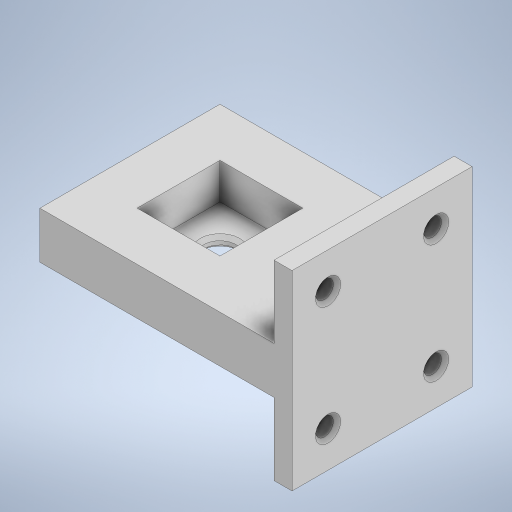
# Autodesk Inventor part: Стенка энкодер
Saved by Autodesk Inventor 2023 (Build 270158000, 158)
## iProperties
Created: 2022-05-02
Part Number: Стенка энкодер
Material: Типовые
Document SubType Name: Modeling
Designer: User
Density: 1 g/cm^3
Appearance: По умолчанию
Author: User
Autodesk Inventor part; units mm, degrees
ref_plane "YZ Plane" through (0, 0, 0) normal (1, 0, 0) x (0, 1, 0)
ref_plane "XZ Plane" through (0, 0, 0) normal (0, 1, 0) x (-1, 0, 0)
ref_plane "XY Plane" through (0, 0, 0) normal (0, 0, 1) x (1, 0, 0)
sketch "Эскиз1" plane through (0, 0, 0) normal (0, 1, 0) x (-1, 0, 0)
  line L0 (0, 0) -> (-70, 0)
  line L1 (-70, 0) -> (-70, -50)
  line L2 (-70, -50) -> (0, -50)
  line L3 (0, -50) -> (0, 0)
  line L4 (-70, 0) -> (-25, 0)
  line L5 (-25, 0) -> (-25, -25)
  line L6 (-25, -25) -> (-70, -25)
  line L7 (-70, -25) -> (-70, 0)
  circle A0 centre (-25, -25) radius 4.5
  dimension "d0" = 70
  dimension "d1" = 50
  dimension "d2" = 45
  dimension "d3" = 25
  dimension "d4" = 9
  constraints: 16 end point, 4 parallel, 2 horizontal, 2 perpendicular, 1 centre point, 1 coincident
  measures "d0" distance of L2.end L1.end
  measures "d1" distance of L1.end L0.end
  measures "d2" distance of L5.end L6.end
  measures "d3" distance of L4.end L5.end
  measures "d4" diameter of A0
extrude "Выдавливание1" add sketch "Эскиз1" along normal blind 3 contours L3 L2 L1 L6 A0 L5 L0 | L5 A0 L6 L1 L0
sketch "Эскиз2" plane through (0, 3, 0) normal (0, 1, 0) x (1, 0, 0)
  circle A0 centre (25, 25) radius 4.5 projected
  line L0 (25, 25) -> (25, 13.5)
  line L1 (25, 13.5) -> (13.5, 13.5)
  line L2 (13.5, 13.5) -> (36.5, 13.5)
  line L3 (36.5, 13.5) -> (36.5, 36.5)
  line L4 (36.5, 36.5) -> (13.5, 36.5)
  line L5 (13.5, 36.5) -> (13.5, 13.5)
  line L6 (70, 50) -> (0, 50) projected
  line L7 (0, 0) -> (70, 0)
  line L8 (70, 0) -> (70, 50)
  line L9 (70, 50) -> (0, 50)
  line L10 (0, 50) -> (0, 0)
  dimension "d7" = 11.5
  dimension "d8" = 11.5
  dimension "d9" = 23
  dimension "d10" = 23
  constraints: 20 end point, 4 parallel, 3 perpendicular, 2 horizontal, 1 vertical
  measures "d7" distance of L0.start L0.end
  measures "d8" distance of L0.end L1.end
  measures "d9" distance of L4.end L3.end
  measures "d10" distance of L3.end L2.end
extrude "Выдавливание2" add sketch "Эскиз2" along normal blind 10 contours L8 L7 L10 L6
sketch "Эскиз3" plane through (70, 0, 0) normal (1, 0, 0) x (0, 0, -1)
  line L0 (0, 0) -> (0, 13) projected
  line L1 (0, 0) -> (0, -20)
  line L2 (0, -20) -> (50, -20)
  line L3 (50, -20) -> (50, 33)
  line L4 (50, 33) -> (0, 33)
  line L5 (0, 33) -> (0, 0)
  line L6 (50, 33) -> (40, 33)
  line L7 (40, 33) -> (40, 23)
  line L8 (0, 33) -> (10, 33)
  line L9 (10, 33) -> (10, 23)
  line L10 (0, -20) -> (10, -20)
  line L11 (10, -20) -> (10, -10)
  line L12 (50, -20) -> (40, -20)
  line L13 (40, -20) -> (40, -10)
  circle A0 centre (40, -10) radius 2.5
  circle A1 centre (10, -10) radius 2.5
  circle A2 centre (10, 23) radius 2.5
  circle A3 centre (40, 23) radius 2.5
  dimension "d13" = 20
  dimension "d14" = 53
  dimension "d15" = 10
  dimension "d16" = 10
  dimension "d17" = 10
  dimension "d18" = 10
  dimension "d19" = 10
  dimension "d20" = 10
  dimension "d21" = 10
  dimension "d22" = 5
  dimension "d23" = 5
  dimension "d24" = 5
  dimension "d25" = 5
  constraints: 26 end point, 7 point on line, 6 perpendicular, 4 centre point, 4 coincident, 1 vertical
  measures "d13" distance of L0.start L1.end
  measures "d14" distance of L2.end L3.end
  measures "d15" distance of L3.end L6.end
  measures "d16" distance of L6.end L7.end
  measures "d17" distance of L4.end L8.end
  measures "d18" distance of L1.end L10.end
  measures "d19" distance of L10.end L11.end
  measures "d20" distance of L2.end L12.end
  measures "d21" distance of L12.end L13.end
  measures "d22" diameter of A0
  measures "d23" diameter of A1
  measures "d24" diameter of A2
  measures "d25" diameter of A3
extrude "Выдавливание3" add sketch "Эскиз3" against normal blind 5
chamfer "Фаска1" distance 1 angle 45 10 edges at (70, -10, -37.5) (70, 23, -37.5) (70, 23, -7.5) (70, -10, -7.5) (29.5, 0, -25) (65, -10, -7.5) (65, -10, -37.5) (29.5, 3, -25) (65, 23, -37.5) (65, 23, -7.5)
